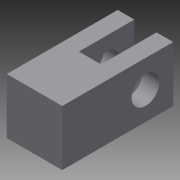
# Autodesk Inventor part: rod grabber
Saved by Autodesk Inventor 2015 (Build 190159000, 159)
## iProperties
Created: 2015-04-10
Part Number: rod grabber
Material: Generic
Document SubType Name: Modeling
Designer: WASHHSST
Density: 1 g/cm^3
Appearance: Default
Author: WASHHSST
Autodesk Inventor part; units mm, degrees
ref_plane "YZ Plane" through (0, 0, 0) normal (1, 0, 0) x (0, 1, 0)
ref_plane "XZ Plane" through (0, 0, 0) normal (0, 1, 0) x (-1, 0, 0)
ref_plane "XY Plane" through (0, 0, 0) normal (0, 0, 1) x (1, 0, 0)
sketch "Sketch1" plane through (0, 0, 0) normal (0, 1, 0) x (-1, 0, 0)
  line L0 (0, 0) -> (12.7, 0)
  line L1 (12.7, 0) -> (12.7, -25.4)
  line L2 (12.7, -25.4) -> (0, -25.4)
  line L3 (0, -25.4) -> (0, 0)
  line L4 (8.89, -25.4) -> (8.89, -12.7)
  line L5 (8.89, -12.7) -> (3.81, -12.7)
  line L6 (3.81, -12.7) -> (3.81, -25.4)
  dimension "d0" = 12.7
  dimension "d1" = 25.4
  dimension "d2" = 3.81
  dimension "d3" = 3.81
  dimension "d4" = 12.7
  constraints: 14 end point, 3 perpendicular, 2 parallel, 2 point on line, 1 horizontal, 1 vertical
  measures "d0" distance of L1.end L2.end
  measures "d1" distance of L0.end L1.end
  measures "d2" distance between parallel lines of L1 L4
  measures "d3" distance between parallel lines of L3 L6
  measures "d4" distance between parallel lines of L2 L5
extrude "Extrusion1" add sketch "Sketch1" along normal blind 12.7 contours L0 L1 L2 L4 L5 L6 L3
hole "Hole1" at (0, 6.35, -19.05) direction (-1, 0, 0) diameter 6.35 end through all
body "Solid1"
